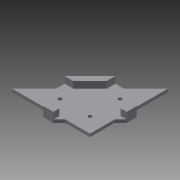
# Autodesk Inventor part: stencil
Saved by Autodesk Inventor 2015 (Build 190159000, 159)
## iProperties
Created: 2017-12-16
Part Number: stencil
Material: Generic
Document SubType Name: Modeling
Designer: Anshul
Density: 1 g/cm^3
Appearance: Default
Author: Anshul
Autodesk Inventor part; units mm, degrees
ref_plane "YZ Plane" through (0, 0, 0) normal (1, 0, 0) x (0, 1, 0)
ref_plane "XZ Plane" through (0, 0, 0) normal (0, 1, 0) x (-1, 0, 0)
ref_plane "XY Plane" through (0, 0, 0) normal (0, 0, 1) x (1, 0, 0)
sketch "Sketch1" plane through (0, 0, 0) normal (0, 1, 0) x (-1, 0, 0)
  line L0 (0, 0) -> (25, 0)
  line L1 (0, -25) -> (0, 0)
  line L2 (25, 0) -> (50, 0)
  circle A0 centre (37.5, -12.5) radius 1.5
  circle A1 centre (12.5, -12.5) radius 1.5
  circle A2 centre (12.5, -37.5) radius 1.5
  line L3 (0, 0) -> (0, -25.5)
  line L4 (50, 0) -> (51, 0)
  line L5 (46.5711, -25.5) -> (39.5, -25.5)
  line L6 (25.5, -39.5) -> (25.5, -46.5711)
  line L7 (0, 0) -> (0, -65)
  line L8 (0, 0) -> (65, 0)
  line L9 (65, 0) -> (0, -65)
  line L10 (25.5, 0) -> (25.5, 5)
  line L11 (25.5, 5) -> (33.9376, 5)
  line L12 (0, -25.5) -> (-5, -25.5)
  line L13 (-5, -25.5) -> (-5, -33.9376)
  line L14 (32.5, -32.5) -> (36.0355, -36.0355)
  line L15 (36.0355, -36.0355) -> (25.5, -46.5711)
  line L16 (36.0355, -36.0355) -> (46.5711, -25.5)
  line L17 (28.9376, 0) -> (33.9376, 5)
  line L18 (-5, -33.9376) -> (0, -28.9376)
  line L19 (12.5, -12.5) -> (12.5, -37.5)
  line L20 (12.5, -12.5) -> (37.5, -12.5)
  line L21 (33.9376, 5) -> (38.9376, 0)
  line L22 (25.5, 5) -> (20.5, 0)
  line L23 (-5, -25.5) -> (0, -20.5)
  line L24 (-5, -33.9376) -> (0, -38.9376)
  line L25 (25.5, -46.5711) -> (18.4289, -46.5711)
  line L26 (46.5711, -25.5) -> (46.5711, -18.4289)
  line L27 (46.5711, -18.4289) -> (39.5, -25.5)
  line L28 (25.5, -39.5) -> (18.4289, -46.5711)
  line L29 (0, -20.5) -> (0, -25.5)
  line L30 (25.5, 0) -> (20.5, 0)
  line L31 (0, -28.9376) -> (0, -38.9376)
  line L32 (0, -20.5) -> (0, -25.5)
  line L33 (0, -25.5) -> (0, -28.9376)
  line L34 (0, -28.9376) -> (0, -38.9376)
  line L35 (-5, -33.9376) -> (0, -38.9376)
  line L36 (0, -38.9376) -> (0, -28.9376)
  line L37 (0, -28.9376) -> (-5, -33.9376)
  dimension "d36" = 25
  dimension "d38" = 25
  dimension "d42" = 3
  dimension "d43" = 3
  dimension "d44" = 3
  dimension "d45" = 25.5
  dimension "d47" = 1
  dimension "d51" = 65
  dimension "d52" = 65
  dimension "d54" = 5
  dimension "d55" = 5
  dimension "d56" = 5
  constraints: 76 end point, 12 perpendicular, 12 point on line, 6 collinear, 6 horizontal, 4 vertical, 3 centre point, 2 parallel, 1 midpoint
  measures "d36" distance of L0.start L0.end
  measures "d38" distance of L0.end L2.end
  measures "d42" diameter of A0
  measures "d43" diameter of A1
  measures "d44" diameter of A2
  measures "d45" distance of L0.start L3.end
  measures "d47" distance of L2.end L4.end
  measures "d51" distance of L0.start L7.end
  measures "d52" distance of L0.start L8.end
  measures "d54" distance of L10.start L10.end
  measures "d55" distance of L3.end L12.end
  measures "d56" distance of L14.start L14.end
extrude "Extrusion5" add sketch "Sketch1" along normal blind 2.5 contours L0 L2 L4 L8 L9 L7 L3 L1 | L22 L10 L2 L0 | L1 L3 L12 L23 | L21 L2 L17 | L18 L7 L24 | L9 L6 L25 | L26 L5 L9
extrude "Extrusion6" add sketch "Sketch1" along normal blind 8 contours L11 L17 L2 L10 | L12 L7 L18 L13 | L9 L14 L15 L6 | L9 L5 L16 L14
body "Solid3"
